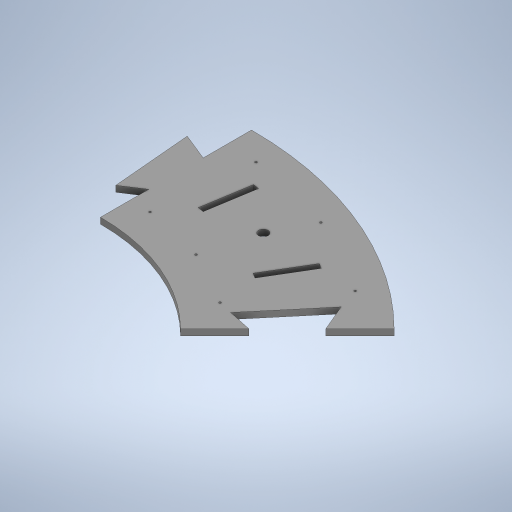
# Autodesk Inventor part: Non-Rotating Carousel Plate
Saved by Autodesk Inventor 2023 (Build 270158000, 158)
## iProperties
Created: 2023-02-13
Part Number: Non-Rotating Carousel Plate
Material: PLA 33 Plastic
Document SubType Name: Modeling
Designer: cheng
Density: 0.4135 g/cm^3
Appearance: Generic
Author: cheng
Autodesk Inventor part; units mm, degrees
ref_plane "YZ Plane" through (0, 0, 0) normal (1, 0, 0) x (0, 1, 0)
ref_plane "XZ Plane" through (0, 0, 0) normal (0, 1, 0) x (-1, 0, 0)
ref_plane "XY Plane" through (0, 0, 0) normal (0, 0, 1) x (1, 0, 0)
sketch "Sketch2" plane through (0, 0, 0) normal (0, 1, 0) x (-1, 0, 0)
  circle A0 centre (0, 0) radius 285
  circle A1 centre (0, 0) radius 160
  line L0 (0, 0) -> (0, -285)
  line L1 (0, 0) -> (-201.5254, -201.5254)
  line L2 (0, 0) -> (24.8394, -283.9155)
  line L3 (0, 0) -> (-183.1945, -218.3227)
  circle A2 centre (0, 0) radius 255
  circle A3 centre (0, 0) radius 190
  circle A4 centre (0, 0) radius 200
  circle A5 centre (0, 0) radius 245
  line L4 (16.5596, -189.277) -> (0, -200)
  line L5 (22.2247, -254.0296) -> (0, -245)
  line L6 (-122.1296, -145.5484) -> (-141.4214, -141.4214)
  line L7 (-163.9108, -195.3413) -> (-173.2412, -173.2412)
  line L8 (-123.7453, -217.2835) -> (-128.0398, -214.7227)
  line L9 (-128.0398, -214.7227) -> (-107.5534, -180.367)
  line L10 (-107.5534, -180.367) -> (-103.2589, -182.9278)
  line L11 (-103.2589, -182.9278) -> (-123.7453, -217.2835)
  line L12 (-123.7453, -217.2835) -> (-107.5534, -180.367) construction
  line L13 (-128.0398, -214.7227) -> (-103.2589, -182.9278) construction
  circle A6 centre (0, 0) radius 230 construction
  line L14 (0, 0) -> (-97.4757, -267.8124) construction
  circle A7 centre (0, 0) radius 210 construction
  circle A8 centre (0, 0) radius 250 construction
  line L15 (-44.8727, -245.9907) -> (-39.9369, -246.7895)
  line L16 (-39.9369, -246.7895) -> (-33.547, -207.3032)
  line L17 (-33.547, -207.3032) -> (-38.4828, -206.5044)
  line L18 (-38.4828, -206.5044) -> (-44.8727, -245.9907)
  line L19 (-44.8727, -245.9907) -> (-33.547, -207.3032) construction
  line L20 (-39.9369, -246.7895) -> (-38.4828, -206.5044) construction
  circle A9 centre (-78.6646, -216.1293) radius 4
  point P0 (-115.6493, -198.8252)
  point P1 (0, -160)
  point P2 (-113.1371, -113.1371)
  dimension "d0" = 570
  dimension "d1" = 320
  dimension "d2" = 45
  dimension "d3" = 5
  dimension "d4" = 5
  dimension "d5" = 30
  dimension "d6" = 30
  dimension "d7" = 10
  dimension "d8" = 10
  dimension "d11" = 5
  dimension "d14" = 20
  dimension "d19" = 39.2099
  dimension "d20" = 40
  dimension "d21" = 50
  dimension "d24" = 8
  dimension "d35" = 70
  constraints: 42 end point, 13 point on circle, 9 centre point, 9 coincident, 9 point on line, 4 symmetric about line, 2 line through centre, 2 parallel, 2 tangent, 1 midpoint, 1 perpendicular, 1 vertical, 3 other
  measures "d0" diameter of A0
  measures "d1" diameter of A1
  measures "d2" angle of L1 L0
  measures "d3" angle of L2 L0
  measures "d4" angle of L1 L3
  measures "d5" radial gap between concentric circles of A0 A2
  measures "d6" radial gap between concentric circles of A3 A1
  measures "d7" radial gap between concentric circles of A3 A4
  measures "d8" radial gap between concentric circles of A5 A2
  measures "d11" distance of L8.start L8.end
  measures "d14" angle of L3 L14
  measures "d19" distance from line of L3 point (-115.649, -198.825)
  measures "d20" radial gap between concentric circles of A8 A7
  measures "d21" radial gap between concentric circles of A1 A7
  measures "d24" diameter of A9
extrude "Extrusion1" add sketch "Sketch2" along normal blind 5 contours L1 A2 L3 A0 | L3 A2 L0 A0 | L1 L7 A2 | L5 A5 L2 | L3 A5 L9 L8 L11 L18 L15 L16 L0 A2 | A5 L0 A4 L2 | A5 L16 L17 L18 L11 L10 L9 L3 A4 L0 | L1 A3 L6 | A4 L4 L2 | A4 L3 A3 L0 | L1 A1 L3 A3 | L3 A1 L0 A3
sketch "Sketch3" plane through (0, 5, 0) normal (0, 1, 0) x (1, 0, 0)
  circle A0 centre (0, 0) radius 185
  circle A1 centre (0, 0) radius 265
  point P0 (94.9402, 247.4093)
  point P1 (66.3297, 172.7002)
  point P2 (16.7015, 184.2446)
  point P3 (24.8728, 263.8301)
  point P4 (110.6548, 148.2583)
  point P5 (158.2673, 212.5475)
  dimension "d32" = 370
  dimension "d34" = 530
  constraints: 6 point on circle, 2 centre point, 2 coincident
  measures "d32" diameter of A0
  measures "d34" diameter of A1
hole "Hole1" at (94.9402, 5, -247.4093) at (66.3297, 5, -172.7002) at (16.7015, 5, -184.2446) at (24.8728, 5, -263.8301) at (110.6548, 5, -148.2583) at (158.2673, 5, -212.5475) direction (0, -1, 0) diameter 1.778 end through all
body "Solid1"
